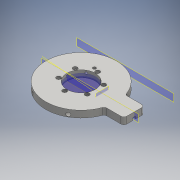
# Autodesk Inventor part: top
Saved by Autodesk Inventor 2016 (Build 200138000, 138)
## iProperties
Created: 2017-05-24
Part Number: top
Material: Generic
Document SubType Name: Modeling
Designer: bitbots
Density: 1 g/cm^3
Appearance: Default
Author: bitbots
Autodesk Inventor part; units mm, degrees
ref_plane "YZ Plane" through (0, 0, 0) normal (1, 0, 0) x (0, 1, 0)
ref_plane "XZ Plane" through (0, 0, 0) normal (0, 1, 0) x (-1, 0, 0)
ref_plane "XY Plane" through (0, 0, 0) normal (0, 0, 1) x (1, 0, 0)
ref_plane "Work Plane1" through (0, 0, 0) normal (0, 0, 1) x (1, 0, 0)
sketch "Sketch1" plane through (0, 0, 0) normal (0, 0, 1) x (1, 0, 0)
  circle A0 centre (7.7356, -42.5713) radius 1.65 construction
  circle A1 centre (7.7356, -14.5713) radius 1.65 construction
  circle A2 centre (-40.7618, -14.5713) radius 1.65 construction
  circle A3 centre (-40.7618, -42.5713) radius 1.65 construction
  circle A4 centre (-16.5131, -56.5713) radius 1.65 construction
  circle A5 centre (-16.5131, -28.5713) radius 23 construction
  circle A6 centre (-16.5131, -0.5713) radius 1.65 construction
  line L0 (8.9285, -4.5354) -> (9.6603, -3.2679) construction
  line L1 (9.6603, -3.2679) -> (-7.1349, 6.4287) construction
  line L2 (-7.1349, 6.4287) -> (-7.8354, 6.4287) construction
  line L3 (-7.8354, 6.4287) -> (-8.3875, 5.4724) construction
  arc A7 (-8.3875, 5.4724) -> (-45.0507, -8.3079) centre (-16.5131, -28.5713) ccw construction
  line L4 (-45.0507, -8.3079) -> (-48.3766, -7.7215) construction
  line L5 (-48.3766, -7.7215) -> (-53.5861, -37.2657) construction
  line L6 (-53.5861, -37.2657) -> (-50.2602, -37.8522) construction
  arc A8 (-50.2602, -37.8522) -> (-45.3149, -48.4574) centre (-16.5131, -28.5713) ccw construction
  line L7 (-45.3149, -48.4574) -> (-47.0035, -51.3822) construction
  line L8 (-47.0035, -51.3822) -> (-25.3528, -63.8822) construction
  line L9 (-25.3528, -63.8822) -> (-24.6234, -62.6186) construction
  arc A9 (-24.6234, -62.6186) -> (8.9285, -4.5354) centre (-16.5131, -28.5713) ccw construction
  circle A10 centre (-16.5131, -28.5713) radius 23
  circle A11 centre (-16.5131, -28.5713) radius 35
  circle A12 centre (-16.5131, -56.5713) radius 1.65
  circle A13 centre (-40.7618, -42.5713) radius 1.65
  circle A14 centre (-40.7618, -14.5713) radius 1.65
  circle A15 centre (-16.5131, -0.5713) radius 1.65
  circle A16 centre (7.7356, -14.5713) radius 1.65
  circle A17 centre (7.7356, -42.5713) radius 1.65
  point P0 (0, 0)
  constraints: 8 centre point, 8 coincident, 8 concentric
extrude "Extrusion1" add sketch "Sketch1" along normal blind 11.5
ref_plane "Work Plane2" through (18.4869, -28.5713, 6.2613) normal (-0.9961947, 0, 0.0871557) x (0, -1, 0)
sketch "Sketch2" plane through (18.4869, -28.5713, 6.2613) normal (-0.9961947, 0, 0.0871557) x (0, -1, 0)
  spline S0 degree 3 poles (-1.3526, 0) (-1.3526, 0.1694) (-1.3188, 0.3504) (-1.1809, 0.6837) (-1.0768, 0.836) (-0.8365, 1.0764) (-0.6844, 1.1805) (-0.3511, 1.3186) (-0.1699, 1.3526) (0.1699, 1.3526) (0.3511, 1.3186) (0.6844, 1.1805) (0.8365, 1.0764) (1.0768, 0.836) (1.1809, 0.6837) (1.3188, 0.3504) (1.3525, 0.1694) (1.3525, -0.1702) (1.3185, -0.3514) (1.1804, -0.6845) (1.0764, -0.8364) (0.8367, -1.0761) (0.685, -1.1801) (0.3518, -1.3184) (0.1704, -1.3525) (-0.1704, -1.3525) (-0.3518, -1.3184) (-0.685, -1.1801) (-0.8367, -1.0761) (-1.0764, -0.8364) (-1.1804, -0.6845) (-1.3185, -0.3514) (-1.3526, -0.1702) (-1.3526, 0) knots 0 0 0 0 0.05101 0.05101 0.10202 0.10202 0.152982 0.152982 0.203944 0.203944 0.254906 0.254906 0.305868 0.305868 0.356878 0.356878 0.407888 0.407888 0.459155 0.459155 0.510422 0.510422 0.561534 0.561534 0.612646 0.612646 0.663758 0.663758 0.71487 0.71487 0.766137 0.766137 0.817404 0.817404 0.817404 0.817404 construction
  circle A0 centre (0, 0) radius 1.8
  point P0 (-28.5713, -7.8487)
  point P1 (-1.3526, 0)
  dimension "d2" = 3.6
  constraints: 1 centre point
  measures "d2" diameter of A0
extrude "Extrusion2" cut sketch "Sketch2" along normal mid plane 30
sketch "Sketch3" plane through (18.4869, -28.5713, 6.2613) normal (-0.9961947, 0, 0.0871557) x (0, -1, 0)
  spline S0 degree 2 poles (1.8, 0) (1.8, 3.1177) (-0.9, 1.5588) (-3.6, 0) (-0.9, -1.5588) (1.8, -3.1177) (1.8, 0) knots 0 0 0 0.333333 0.333333 0.666667 0.666667 1 1 1 weights 1 0.5 1 0.5 1 0.5 1 projected
  circle A0 centre (0, 0) radius 3.15
  point P0 (-28.5713, -7.8487)
  dimension "d5" = 6.3
  constraints: 1 centre point, 1 other
  measures "d5" diameter of A0
extrude "Extrusion3" cut sketch "Sketch3" along normal mid plane 6
pattern_circular "Circular Pattern1" count 6 over 360 about axis through (-16.5131, -28.5713, 0) along (0, 0, 1) of "Extrusion3", "Extrusion2"
ref_plane "Work Plane3" through (-16.5131, -28.5713, 2.5) normal (0, 0, -1) x (-1, 0, 0)
sketch "Sketch4" plane through (-16.5131, -28.5713, 2.5) normal (0, 0, -1) x (-1, 0, 0)
  line L0 (2.7846, -43.1769) -> (-38.7846, -19.1769) projected
  line L1 (2.7846, -43.1769) -> (-5.2154, -57.0333) projected
  line L2 (-46.7846, -33.0333) -> (-5.2154, -57.0333) projected
  line L3 (-38.7846, -19.1769) -> (-46.7846, -33.0333) projected
  circle A0 centre (0, 0) radius 35 projected
  line L4 (2.7846, -43.1769) -> (8.0469, -34.0624)
  line L5 (-38.7846, -19.1769) -> (-33.5223, -10.0624)
  line L6 (8.0469, -34.0624) -> (-17.5, -30.3109)
  line L7 (-17.5, -30.3109) -> (-33.5223, -10.0624)
  point P0 (-16.5131, 28.5713)
  constraints: 8 end point, 3 point on circle, 1 parallel
extrude "Extrusion4" add sketch "Sketch4" against normal blind 2 contours L1 L2 L3 L0 | L0 L5 A0 L4
ref_plane "Work Plane4" through (-16.5131, -28.5713, 7) normal (0, 0, -1) x (-1, 0, 0)
sketch "Sketch5" plane through (-16.5131, -28.5713, 7) normal (0, 0, -1) x (-1, 0, 0)
  line L0 (-36, -4) -> (-87, -4) projected
  line L1 (-36, -4) -> (-36, -14) projected
  line L2 (-87, -14) -> (-36, -14) projected
  line L3 (-87, -4) -> (-87, -14) projected
  line L4 (8.0469, -34.0624) -> (-5.2154, -57.0333) projected
  line L5 (-5.2154, -57.0333) -> (-46.7846, -33.0333) projected
  line L6 (-46.7846, -33.0333) -> (-33.5223, -10.0624) projected
  arc A0 (-33.5223, -10.0624) -> (-19.7119, -28.9213) centre (0, 0) ccw projected
  arc A1 (-19.7119, -28.9213) -> (-15.1906, -31.5317) centre (0, 0) ccw projected
  arc A2 (-15.1906, -31.5317) -> (8.0469, -34.0624) centre (0, 0) ccw projected
  circle A3 centre (0, 0) radius 35 projected
  line L7 (-87, -4) -> (-87, 0)
  line L8 (29.1046, -46.4106) -> (37.7648, -41.4106) projected
  line L9 (38.7648, -43.1426) -> (37.7648, -41.4106) projected
  arc A4 (38.7648, -43.1426) -> (58, 0.0727) centre (0, 0) ccw projected
  line L10 (58, 0.0727) -> (56.0303, -0.2746) projected
  line L11 (56.0303, -0.2746) -> (52.5574, 19.4215) projected
  line L12 (54.527, 19.7688) -> (52.5574, 19.4215) projected
  arc A5 (54.527, 19.7688) -> (11.225, 56.9034) centre (0, 0) ccw projected
  line L13 (11.225, 58.9406) -> (11.225, 56.9034) projected
  arc A6 (-56.2907, -20.7692) -> (11.225, 58.9406) centre (0, 0) ccw construction
  arc A7 (-56.2907, -20.7692) -> (-60.9816, -17.5) centre (-60.9816, -22.5) ccw projected
  line L14 (-85, -17.5) -> (-60.9816, -17.5) projected
  arc A8 (-90, -12.5) -> (-85, -17.5) centre (-85, -12.5) ccw projected
  line L15 (-90, 0) -> (-90, -12.5) projected
  line L16 (-88, 0) -> (-90, 0) projected
  line L17 (-88, -10.5) -> (-88, 0) projected
  arc A9 (-88, -10.5) -> (-83, -15.5) centre (-83, -10.5) ccw projected
  line L18 (-42.5, -15.5) -> (-83, -15.5) projected
  line L19 (-42.5, -15.5) -> (-42.5, -19.5) projected
  line L20 (-42.5, -19.5) -> (-54.6237, -19.5) projected
  arc A10 (-54.6237, -19.5) -> (-51.3747, -26.9191) centre (0, 0) ccw projected
  line L21 (-51.3747, -26.9191) -> (-45.7176, -30.1852) projected
  line L22 (-45.7176, -30.1852) -> (-47.2176, -32.7833) projected
  line L23 (-47.2176, -32.7833) -> (-4.7824, -57.2833) projected
  line L24 (-4.7824, -57.2833) -> (-3.2824, -54.6852) projected
  line L25 (-3.2824, -54.6852) -> (2.3747, -57.9514) projected
  arc A11 (2.3747, -57.9514) -> (30.7148, -49.1996) centre (0, 0) ccw projected
  line L26 (30.7148, -49.1996) -> (29.1046, -46.4106) projected
  line L27 (-60.9816, -17.5) -> (-60.9816, -15.5)
  line L28 (-60.9816, -15.5) -> (-83, -15.5)
  line L29 (-90, 0) -> (-87, 0)
  line L30 (-87, -4) -> (-90, -4)
  line L31 (-90, -4) -> (-90, 0)
  line L32 (-88, -4) -> (-29.7606, -4)
  line L33 (-29.7606, -4) -> (-29.7606, -15.5)
  line L34 (-29.7606, -15.5) -> (-88, -15.5)
  line L35 (-88, -15.5) -> (-88, -4)
  line L36 (-54.6237, -19.5) -> (-35.2604, -19.5)
  line L37 (-35.2604, -19.5) -> (-35.2604, -15.5)
  line L38 (-35.2604, -15.5) -> (-54.6237, -15.5)
  line L39 (-54.6237, -15.5) -> (-54.6237, -19.5)
  line L40 (-47.9586, -33.5041) -> (-35.2604, -33.5041)
  line L41 (-35.2604, -33.5041) -> (-35.2604, -19.5)
  line L42 (-35.2604, -19.5) -> (-47.9586, -19.5)
  line L43 (-47.9586, -19.5) -> (-47.9586, -33.5041)
  line L44 (-47.9586, -19.5) -> (-51.9058, -19.5)
  line L45 (-51.9058, -19.5) -> (-51.9058, -28.939)
  line L46 (-51.9058, -28.939) -> (-47.9586, -28.939)
  line L47 (-47.9586, -28.939) -> (-47.9586, -19.5)
  line L48 (-51.9058, -19.5) -> (-53.3897, -19.5)
  line L49 (-53.3897, -19.5) -> (-53.3897, -26.2863)
  line L50 (-53.3897, -26.2863) -> (-51.9058, -26.2863)
  line L51 (-51.9058, -26.2863) -> (-51.9058, -19.5)
  line L52 (-53.3897, -19.5) -> (-55.0309, -19.5)
  line L53 (-55.0309, -19.5) -> (-55.0309, -22.8932)
  line L54 (-55.0309, -22.8932) -> (-53.3897, -22.8932)
  line L55 (-53.3897, -22.8932) -> (-53.3897, -19.5)
  line L56 (-3.2824, -54.6852) -> (8.7201, -33.8963)
  line L57 (8.7201, -33.8963) -> (8.4423, -33.3775)
  line L58 (8.0469, -34.0624) -> (-5.2154, -57.0333) projected
  line L59 (8.4423, -33.3775) -> (8.0469, -34.0624)
  line L60 (8.0469, -34.0624) -> (-5.2154, -57.0333)
  line L61 (-5.2154, -57.0333) -> (-4.7824, -57.2833)
  line L62 (-3.2824, -54.6852) -> (-4.7824, -57.2833)
  line L63 (-4.7824, -57.2833) -> (-6.1674, -59.6822)
  arc A12 (-56.2907, -20.7692) -> (-6.1674, -59.6822) centre (0, 0) ccw
  line L64 (-47.2176, -32.7833) -> (-47.2176, -21.5468)
  line L65 (-47.2176, -21.5468) -> (-54.6237, -15.5)
  line L66 (-54.6237, -15.5) -> (-60.9816, -15.5)
  point P0 (-16.5131, 28.5713)
  dimension "d15" = 4
  constraints: 80 end point, 13 parallel, 11 perpendicular, 7 point on line, 6 horizontal, 4 point on circle, 3 collinear, 1 centre point, 1 coincident, 1 tangent, 1 vertical
  measures "d15" distance of L0.end L7.end
extrude "Extrusion5" add sketch "Sketch5" against normal blind 2 contours L1 L2 A9 L3 L0 | L32 A3 L6 L34 L18 A9 L2 L1 | L3 A9 L17 L30 | L32 L33 L34 A0 A3 | A9 L2 L3 | L3 L2 A9 L34 L35 | L17 L35 L34 L18 L27 L14 A8 L15 L30 | A0 L34 L6 | L56 L24 L23 L4 A3 | A3 L59 L57 | L34 L37 L36 L6 | L6 L36 L19 L34 | A0 A1 A2 L4 L5 L40 L41 L37 L34 | L18 L39 L52 L53 L54 L49 L50 L45 L46 L43 L40 L5 L23 L63 A12 A7 L27 | L36 L41 L40 L5 L6 | L6 L23 L22 L21 L64 L65 L43 L20 L36 | L19 L20 L65 L18 | L65 L20 L39 | L5 L40 L43 L21 L64 L23 | L20 L49 A10 | A10 L49 L54 L53 L52 | L65 L43 L21 A10 L45 L20 | L20 L43 L65 | L64 L21 L22 | L20 L45 A10 L49 | A10 L45 L50 L49 | L65 L64 L21 L43 | A10 L21 L43 L46 L45
sketch "Sketch6" plane through (-16.5131, -28.5713, 4.5) normal (0, 0, 1) x (1, 0, 0)
  line L0 (-8.0469, -34.0624) -> (5.2154, -57.0333) projected
  line L1 (5.2154, -57.0333) -> (46.7846, -33.0333) projected
  line L2 (46.7846, -33.0333) -> (33.5223, -10.0624) projected
  arc A0 (19.7119, -28.9213) -> (33.5223, -10.0624) centre (0, 0) ccw projected
  arc A1 (15.1906, -31.5317) -> (19.7119, -28.9213) centre (0, 0) ccw projected
  arc A2 (-8.0469, -34.0624) -> (15.1906, -31.5317) centre (0, 0) ccw projected
  point P0 (16.5131, 28.5713)
extrude "Extrusion6" add sketch "Sketch6" along normal up to surface (2.5 mm away)
sketch "Sketch7" plane through (-16.5131, -28.5713, 11.5) normal (0, 0, 1) x (1, 0, 0)
  arc A0 (-11.225, 58.9406) -> (56.2907, -20.7692) centre (0, 0) ccw construction
  arc A1 (-8.7201, -33.8963) -> (34.7707, -4) centre (0, 0) ccw projected
  circle A2 centre (0, 0) radius 35
  arc A3 (90, 12.5) -> (85, 17.5) centre (85, 12.5) ccw projected
  line L0 (90, 12.5) -> (90, -12.5) projected
  arc A4 (85, -17.5) -> (90, -12.5) centre (85, -12.5) ccw projected
  line L1 (85, -17.5) -> (60.9816, -17.5) projected
  arc A5 (60.9816, -17.5) -> (56.2907, -20.7692) centre (60.9816, -22.5) ccw projected
  arc A6 (56.2907, 20.7692) -> (56.2907, -20.7692) centre (0, 0) ccw construction
  arc A7 (56.2907, 20.7692) -> (60.9816, 17.5) centre (60.9816, 22.5) ccw projected
  line L2 (60.9816, 17.5) -> (85, 17.5) projected
  circle A8 centre (0, 0) radius 33 construction
  arc A9 (56.2907, 20.7692) -> (56.2907, -20.7692) centre (0, 0) ccw
  point P0 (16.5131, 28.5713)
  constraints: 2 centre point, 2 coincident, 2 point on circle
extrude "Extrusion7" add sketch "Sketch7" against normal up to surface (4.5 mm away)
sketch "Sketch8" plane through (0, 0, 11.5) normal (0, 0, 1) x (1, 0, 0)
  circle A0 centre (7.7356, -42.5713) radius 1.65 projected
  circle A1 centre (7.7356, -42.5713) radius 3.1
  arc A2 (-47.8124, -39.0285) -> (15.6233, -36.0713) centre (-16.5131, -28.5713) ccw projected
  arc A3 (44.4685, -46.0713) -> (39.7776, -49.3405) centre (44.4685, -51.0713) ccw projected
  line L0 (44.4685, -46.0713) -> (68.4869, -46.0713) projected
  arc A4 (68.4869, -46.0713) -> (73.4869, -41.0713) centre (68.4869, -41.0713) ccw projected
  line L1 (73.4869, -41.0713) -> (73.4869, -16.0713) projected
  arc A5 (73.4869, -16.0713) -> (68.4869, -11.0713) centre (68.4869, -16.0713) ccw projected
  line L2 (68.4869, -11.0713) -> (44.4685, -11.0713) projected
  arc A6 (39.7776, -7.802) -> (44.4685, -11.0713) centre (44.4685, -6.0713) ccw projected
  arc A7 (39.7776, -7.802) -> (39.7776, -49.3405) centre (-16.5131, -28.5713) ccw projected
  circle A8 centre (-16.5131, -28.5713) radius 23 projected
  circle A9 centre (7.7356, -42.5713) radius 1.65 projected
  circle A10 centre (7.7356, -14.5713) radius 1.65 projected
  circle A11 centre (-16.5131, -0.5713) radius 1.65 projected
  circle A12 centre (-40.7618, -14.5713) radius 1.65 projected
  circle A13 centre (-40.7618, -42.5713) radius 1.65 projected
  circle A14 centre (-16.5131, -56.5713) radius 1.65 projected
  circle A15 centre (7.7356, -14.5713) radius 3.1
  circle A16 centre (-16.5131, -0.5713) radius 3.1
  circle A17 centre (-40.7618, -14.5713) radius 3.1
  circle A18 centre (-40.7618, -42.5713) radius 3.1
  circle A19 centre (-16.5131, -56.5713) radius 3.1
  point P0 (0, 0)
  dimension "d22" = 6.2
  dimension "d25" = 360
  constraints: 6 centre point, 1 coincident, 13 other
  measures "d22" diameter of A1
extrude "Extrusion8" cut sketch "Sketch8" against normal blind 3.5 contours A1 | A10 | A15 | A16 | A17 | A18 | A19
sketch "Sketch9" plane through (-16.5131, -28.5713, 7) normal (0, 0, -1) x (-1, 0, 0)
  line L0 (-90, 12.5) -> (-90, -12.5) construction
  arc A0 (-90, -12.5) -> (-85, -17.5) centre (-85, -12.5) ccw construction
  line L1 (-85, -17.5) -> (-60.9816, -17.5) construction
  arc A1 (-56.2907, -20.7692) -> (-60.9816, -17.5) centre (-60.9816, -22.5) ccw construction
  arc A2 (-56.2907, -20.7692) -> (-56.2907, 20.7692) centre (0, 0) ccw construction
  arc A3 (-60.9816, 17.5) -> (-56.2907, 20.7692) centre (-60.9816, 22.5) ccw construction
  line L2 (-60.9816, 17.5) -> (-85, 17.5) projected
  arc A4 (-85, 17.5) -> (-90, 12.5) centre (-85, 12.5) ccw projected
  arc A5 (-34.8655, -3.0656) -> (-33.5223, -10.0624) centre (0, 0) ccw construction
  arc A6 (-34.8655, 3.0656) -> (-34.8655, -3.0656) centre (0, 0) ccw construction
  arc A7 (-20.0876, 28.6616) -> (-34.8655, 3.0656) centre (0, 0) ccw construction
  arc A8 (-14.7778, 31.7272) -> (-20.0876, 28.6616) centre (0, 0) ccw construction
  arc A9 (14.7778, 31.7272) -> (-14.7778, 31.7272) centre (0, 0) ccw construction
  arc A10 (20.0876, 28.6616) -> (14.7778, 31.7272) centre (0, 0) ccw construction
  arc A11 (34.8655, 3.0656) -> (20.0876, 28.6616) centre (0, 0) ccw construction
  arc A12 (34.8655, -3.0656) -> (34.8655, 3.0656) centre (0, 0) ccw construction
  arc A13 (20.0876, -28.6616) -> (34.8655, -3.0656) centre (0, 0) ccw construction
  arc A14 (14.7778, -31.7272) -> (20.0876, -28.6616) centre (0, 0) ccw construction
  arc A15 (8.0469, -34.0624) -> (14.7778, -31.7272) centre (0, 0) ccw construction
  line L3 (8.0469, -34.0624) -> (-5.2154, -57.0333) construction
  line L4 (-5.2154, -57.0333) -> (-46.7846, -33.0333) construction
  line L5 (-46.7846, -33.0333) -> (-33.5223, -10.0624) construction
  line L6 (-90, -12.5) -> (-90, 12.5) projected
  line L7 (-90, 0) -> (-35, 0)
  circle A16 centre (0, 0) radius 35 projected
  line L8 (8.0469, -34.0624) -> (8.0469, -59.458)
  arc A17 (-56.2907, -20.7692) -> (-56.2907, 20.7692) centre (0, 0) ccw projected
  line L9 (8.0469, -34.0624) -> (33.4424, -34.0624) construction
  arc A18 (8.0469, -34.0624) -> (-35, 0) centre (0, 0) ccw
  arc A19 (-60.9816, 17.5) -> (-56.2907, 20.7692) centre (-60.9816, 22.5) ccw projected
  arc A20 (8.0469, -59.458) -> (-56.2907, 20.7692) centre (0, 0) ccw
  line L10 (-90, 12.5) -> (-90, -12.5) projected
  line L11 (-90, 0) -> (-90, 12.5)
  line L12 (-5.2154, -57.0333) -> (8.0469, -34.0624) projected
  arc A21 (-33.5223, -10.0624) -> (8.0469, -34.0624) centre (0, 0) ccw projected
  line L13 (-33.5223, -10.0624) -> (-46.7846, -33.0333) projected
  line L14 (-46.7846, -33.0333) -> (-5.2154, -57.0333) projected
  line L15 (-46.7846, -33.0333) -> (-5.2154, -57.0333) projected
  line L16 (-46.7846, -33.0333) -> (-48.2801, -35.6235)
  arc A22 (-56.2907, -20.7692) -> (-56.2907, 20.7692) centre (0, 0) ccw projected
  line L17 (-46.7846, -33.0333) -> (-43.7937, -33.0333) construction
  arc A23 (-48.2801, -35.6235) -> (8.0469, -59.458) centre (0, 0) ccw
  line L18 (-5.2154, -57.0333) -> (8.0469, -34.0624) projected
  line L19 (-46.7846, -33.0333) -> (-5.2154, -57.0333)
  line L20 (-5.2154, -57.0333) -> (8.0469, -34.0624)
  arc A24 (-48.2801, -35.6235) -> (8.0469, -59.458) centre (0, 0) ccw
  line L21 (-48.2801, -35.6235) -> (-46.7846, -33.0333)
  line L22 (-46.7846, -33.0333) -> (-5.2154, -57.0333)
  line L23 (-5.2154, -57.0333) -> (8.0469, -34.0624)
  point P0 (-16.5131, 28.5713)
  dimension "d29" = 90
  dimension "d32" = 120
  constraints: 22 end point, 11 point on circle, 4 centre point, 4 coincident, 2 collinear, 2 equal length, 2 horizontal, 2 perpendicular, 1 midpoint, 1 vertical, 2 other
  measures "d29" angle of L8 L9
  measures "d32" angle of L16 L17
extrude "Extrusion9" add sketch "Sketch9" along normal blind 7 contours A19 A17 L8 A16 L7 L6 A4 L2 | A17 L16 L14 L12 L8
sketch "Sketch10" plane through (0, 0, 0) normal (0, 0, -1) x (-1, 0, 0)
  line L0 (-31.767, -64.1948) -> (-17.0093, -38.6337) construction
  arc A0 (-18.3524, -31.6369) -> (-17.0093, -38.6337) centre (16.5131, -28.5713) ccw construction
  arc A1 (-18.4869, -28.5713) -> (-18.3524, -31.6369) centre (16.5131, -28.5713) ccw construction
  line L1 (-18.4869, -28.5713) -> (-73.4869, -28.5713) construction
  line L2 (-73.4869, -28.5713) -> (-73.4869, -41.0713) projected
  arc A2 (-73.4869, -41.0713) -> (-68.4869, -46.0713) centre (-68.4869, -41.0713) ccw projected
  line L3 (-68.4869, -46.0713) -> (-44.4685, -46.0713) projected
  arc A3 (-39.7776, -49.3405) -> (-44.4685, -46.0713) centre (-44.4685, -51.0713) ccw projected
  arc A4 (-39.7776, -49.3405) -> (-31.767, -64.1948) centre (16.5131, -28.5713) ccw projected
  line L4 (11.2977, -85.6046) -> (-30.2715, -61.6046) construction
  line L5 (-30.2715, -61.6046) -> (-31.767, -64.1948) projected
  line L6 (-31.767, -64.1948) -> (-30.2715, -61.6046)
  line L7 (-73.4869, -28.5713) -> (-71.4869, -28.5713)
  line L8 (-71.4869, -28.5713) -> (-71.4869, -41.2625)
  line L9 (-44.4685, -46.0713) -> (-68.4869, -46.0713) projected
  line L10 (-68.4869, -46.0713) -> (-68.4869, -44.0713)
  line L11 (-68.4869, -44.0713) -> (-71.4869, -41.2625)
  arc A5 (-38.6208, -44.0713) -> (-30.2715, -61.6046) centre (16.5131, -28.5713) ccw
  line L12 (-38.6208, -44.0713) -> (-68.4869, -44.0713)
  point P0 (0, 0)
  dimension "d33" = 2
  dimension "d34" = 2
  constraints: 12 end point, 2 point on circle, 1 centre point, 1 coincident, 1 collinear, 1 horizontal, 1 perpendicular, 1 point on line, 1 vertical
  measures "d33" distance of L1.end L7.end
  measures "d34" distance of L3.start L10.end
extrude "Extrusion10" add sketch "Sketch10" against normal up to surface (7 mm away)
sketch "Sketch11" plane through (15.4983, -28.5713, 6.5227) normal (0.9961947, 0, -0.0871557) x (-0.0871557, 0, -0.9961947)
  circle A0 centre (0, 0) radius 1.8 projected
  circle A1 centre (0, 0) radius 3.15 projected
  point P0 (7.8487, 28.5713)
extrude "Extrusion11" cut sketch "Sketch11" along normal blind 100 contours A0 | A1
pattern_circular "Circular Pattern2" count 6 over 360 about axis through (-16.5131, -28.5713, 0) along (0, 0, 1) of "Extrusion11"
ref_plane "Work Plane6" through (44.4685, 31.4287, 11.5) normal (0, 1, 0) x (1, 0, 0)
ref_plane "Work Plane5" through (44.4685, -28.5713, 11.5) normal (0, 1, 0) x (1, 0, 0)
sketch "Sketch12" plane through (44.4685, 31.4287, 11.5) normal (0, 1, 0) x (1, 0, 0)
  spline S0 degree 3 poles (-73.4816, 17) (-73.4816, 18.5746) (-73.1659, 20.2508) (-71.8889, 23.3291) (-70.9276, 24.7316) (-68.7132, 26.946) (-67.3107, 27.9073) (-64.2323, 29.1844) (-62.556, 29.5) (-59.4071, 29.5) (-57.7308, 29.1844) (-54.6524, 27.9073) (-53.2499, 26.946) (-51.0355, 24.7316) (-50.0743, 23.3291) (-48.7972, 20.2508) (-48.4816, 18.5746) (-48.4816, 15.4254) (-48.7972, 13.7492) (-49.5353, 11.97) (-49.6424, 11.733) (-49.7566, 11.5) knots 0 0 0 0 0.472366 0.472366 0.944732 0.944732 1.417066 1.417066 1.8894 1.8894 2.361735 2.361735 2.834069 2.834069 3.306435 3.306435 3.778801 3.778801 4.251167 4.251167 4.324846 4.324846 4.324846 4.324846 projected
  spline S1 degree 3 poles (-72.2065, 11.5) (-72.3207, 11.733) (-72.4278, 11.97) (-73.1659, 13.7492) (-73.4816, 15.4254) (-73.4816, 17) knots 7.011557 7.011557 7.011557 7.011557 7.085236 7.085236 7.557602 7.557602 7.557602 7.557602 projected
  line L0 (-120.9816, 0) -> (-4.6909, 0) construction
  line L1 (-4.6909, 11.5) -> (-120.9816, 11.5) construction
  line L2 (-37.9816, 0) -> (-83.9816, 0) construction
  line L3 (-60.9816, 0) -> (-60.9816, 17) construction
  line L4 (-60.9816, 0) -> (-43.9816, 0) construction
  circle A0 centre (-60.9816, 17) radius 12.4991
  point P0 (-44.4685, 11.5)
  dimension "d43" = 17
  dimension "d44" = 90
  constraints: 4 end point, 1 centre point, 1 coincident, 1 horizontal, 1 midpoint, 1 perpendicular, 1 vertical
  measures "d43" distance of L3.start L3.end
  measures "d44" angle of L4 L3
extrude "Extrusion12" cut sketch "Sketch12" against normal blind 10
sketch "Sketch13" plane through (0, 0, 11.5) normal (0, 0, 1) x (1, 0, 0)
  circle A0 centre (-24.7306, 2.0969) radius 2.3939 construction
  circle A1 centre (-24.7306, 2.0969) radius 2.6
  point P0 (0, 0)
  dimension "d47" = 5.2
  constraints: 1 centre point, 1 coincident
  measures "d47" diameter of A1
extrude "Extrusion13" cut sketch "Sketch13" against normal blind 10
sketch "Sketch14" plane through (0, 0, 0) normal (0, 0, -1) x (-1, 0, 0)
  circle A0 centre (40.7618, -14.5713) radius 1.65 construction
  circle A1 centre (40.7618, -14.5713) radius 2.15
  point P0 (0, 0)
  dimension "d50" = 4.3
  constraints: 1 centre point, 1 coincident
  measures "d50" diameter of A1
extrude "Extrusion14" cut sketch "Sketch14" against normal through all
pattern_circular "Circular Pattern3" count 6 over 360 about axis through (-16.5131, -28.5713, 0) along (0, 0, 1) of "Extrusion14"
sketch "Sketch15" plane through (0, 0, 11.5) normal (0, 0, 1) x (1, 0, 0)
  circle A0 centre (-40.7618, -14.5713) radius 3.1 projected
  circle A1 centre (-40.7618, -14.5713) radius 3.65
  point P0 (0, 0)
  dimension "d56" = 7.3
  constraints: 1 centre point, 1 coincident
  measures "d56" diameter of A1
extrude "Extrusion15" cut sketch "Sketch15" against normal up to surface (3.5 mm away)
pattern_circular "Circular Pattern4" count 6 over 360 about axis through (-16.5131, -28.5713, 0) along (0, 0, 1) of "Extrusion15"
sketch "Sketch17" plane through (0, 0, 0) normal (0, 0, -1) x (-1, 0, 0)
  circle A0 centre (16.5131, -0.5713) radius 2.15 projected
  circle A1 centre (-7.7356, -14.5713) radius 2.15 projected
  circle A2 centre (-7.7356, -42.5713) radius 2.15 projected
  circle A3 centre (16.5131, -56.5713) radius 2.15 projected
  circle A4 centre (40.7618, -42.5713) radius 2.15 projected
  circle A5 centre (40.7618, -14.5713) radius 2.15 projected
  circle A6 centre (16.5131, -28.5713) radius 23 projected
  line L0 (27.7371, 30.3696) -> (27.7371, 21.4287) projected
  line L1 (27.7371, 21.4287) -> (5.2891, 21.4287) projected
  line L2 (5.2891, 21.4287) -> (5.2891, 30.3696) projected
  arc A7 (5.2891, 30.3696) -> (-39.7776, -7.802) centre (16.5131, -28.5713) ccw projected
  arc A8 (-44.4685, -11.0713) -> (-39.7776, -7.802) centre (-44.4685, -6.0713) ccw projected
  line L3 (-44.4685, -11.0713) -> (-68.4869, -11.0713) projected
  arc A9 (-68.4869, -11.0713) -> (-73.4869, -16.0713) centre (-68.4869, -16.0713) ccw projected
  line L4 (-73.4869, -16.0713) -> (-73.4869, -25.7717) projected
  ellipse E0 centre (-90.0533, -28.5713) end of major axis (-126.1955, -28.5713) minor radius 3.15 (-53.9112, -28.5713) -> (-73.4869, -25.7717) ccw projected
  line L5 (-53.9112, -28.5713) -> (-18.4869, -28.5713) projected
  arc A10 (-18.4869, -28.5713) -> (24.56, -62.6337) centre (16.5131, -28.5713) ccw projected
  line L6 (24.56, -62.6337) -> (11.2977, -85.6046) projected
  line L7 (11.2977, -85.6046) -> (-30.2715, -61.6046) projected
  arc A11 (-38.6208, -44.0713) -> (-30.2715, -61.6046) centre (16.5131, -28.5713) ccw projected
  line L8 (-38.6208, -44.0713) -> (-68.4869, -44.0713) projected
  line L9 (-68.4869, -44.0713) -> (-71.4869, -41.2625) projected
  line L10 (-71.4869, -41.2625) -> (-71.4869, -31.2739) projected
  ellipse E1 centre (-90.0533, -28.5713) end of major axis (-126.1955, -28.5713) minor radius 3.15 (-73.4869, -31.3709) -> (-71.4869, -31.2739) ccw projected
  line L11 (-73.4869, -31.3709) -> (-73.4869, -41.0713) projected
  arc A12 (-73.4869, -41.0713) -> (-68.4869, -46.0713) centre (-68.4869, -41.0713) ccw projected
  line L12 (-68.4869, -46.0713) -> (-44.4685, -46.0713) projected
  arc A13 (-39.7776, -49.3405) -> (-44.4685, -46.0713) centre (-44.4685, -51.0713) ccw projected
  arc A14 (-39.7776, -49.3405) -> (27.7371, 30.3696) centre (16.5131, -28.5713) ccw projected
  arc A15 (-39.7776, -49.3405) -> (-39.7776, -7.802) centre (16.5131, -28.5713) ccw projected
  arc A16 (45.5131, 21.6582) -> (16.5131, 29.4287) centre (16.5131, -28.5713) ccw
  line L13 (16.5131, -28.5713) -> (16.5131, 29.4287) construction
  line L14 (16.5131, -28.5713) -> (74.5131, -28.5713) construction
  line L15 (16.5131, -28.5713) -> (45.5131, 21.6582) construction
  arc A17 (16.5131, 29.4287) -> (-12.4869, 21.6582) centre (16.5131, -28.5713) ccw
  line L16 (16.5131, -28.5713) -> (-12.4869, 21.6582) construction
  line L17 (16.5131, -28.5713) -> (16.5131, 29.4287) construction
  arc A18 (41.5131, 14.73) -> (16.5131, 21.4287) centre (16.5131, -28.5713) ccw
  line L18 (16.5131, -28.5713) -> (16.5131, 21.4287) construction
  line L19 (16.5131, -28.5713) -> (66.5131, -28.5713) construction
  arc A19 (16.5131, 21.4287) -> (-8.4869, 14.73) centre (16.5131, -28.5713) ccw
  line L20 (16.5131, -28.5713) -> (-8.4869, 14.73) construction
  line L21 (16.5131, -28.5713) -> (16.5131, 21.4287) construction
  line L22 (45.5131, 21.6582) -> (41.5131, 14.73)
  line L23 (-8.4869, 14.73) -> (-12.4869, 21.6582)
  dimension "d72" = 58
  dimension "d73" = 90
  dimension "d74" = 30
  dimension "d75" = 30
  dimension "d76" = 50
  dimension "d77" = 90
  dimension "d78" = 30
  constraints: 22 end point, 8 point on circle, 4 centre point, 4 coincident, 2 horizontal, 2 perpendicular, 1 collinear, 2 other
  measures "d72" radius of A16
  measures "d73" angle of L14 L13
  measures "d74" angle of L15 L13
  measures "d75" angle of L17 L16
  measures "d76" radius of A18
  measures "d77" angle of L19 L18
  measures "d78" angle of L21 L20
extrude "Extrusion17" cut sketch "Sketch17" against normal blind 9.5 contours A16 L22 A18 L1 L0 | L0 L1 L2 A17 A16 | L2 L1 A19 L23 A17
sketch "Sketch16" plane through (0, 0, 0) normal (0, 0, -1) x (-1, 0, 0)
  circle A0 centre (16.5131, -0.5713) radius 2.15 projected
  circle A1 centre (-7.7356, -14.5713) radius 2.15 projected
  circle A2 centre (-7.7356, -42.5713) radius 2.15 projected
  circle A3 centre (16.5131, -56.5713) radius 2.15 projected
  circle A4 centre (40.7618, -42.5713) radius 2.15 projected
  circle A5 centre (40.7618, -14.5713) radius 2.15 projected
  circle A6 centre (16.5131, -28.5713) radius 23 projected
  line L0 (27.7371, 30.3696) -> (27.7371, 28.3323) projected
  line L1 (5.2891, 28.3323) -> (5.2891, 30.3696) projected
  arc A7 (5.2891, 30.3696) -> (-39.7776, -7.802) centre (16.5131, -28.5713) ccw projected
  arc A8 (-44.4685, -11.0713) -> (-39.7776, -7.802) centre (-44.4685, -6.0713) ccw projected
  line L2 (-44.4685, -11.0713) -> (-68.4869, -11.0713) projected
  arc A9 (-68.4869, -11.0713) -> (-73.4869, -16.0713) centre (-68.4869, -16.0713) ccw projected
  line L3 (-73.4869, -16.0713) -> (-73.4869, -25.7717) projected
  ellipse E0 centre (-90.0533, -28.5713) end of major axis (-126.1955, -28.5713) minor radius 3.15 (-53.9112, -28.5713) -> (-73.4869, -25.7717) ccw projected
  line L4 (-53.9112, -28.5713) -> (-18.4869, -28.5713) projected
  arc A10 (-18.4869, -28.5713) -> (24.56, -62.6337) centre (16.5131, -28.5713) ccw projected
  line L5 (24.56, -62.6337) -> (11.2977, -85.6046) projected
  line L6 (11.2977, -85.6046) -> (-30.2715, -61.6046) projected
  arc A11 (-38.6208, -44.0713) -> (-30.2715, -61.6046) centre (16.5131, -28.5713) ccw projected
  line L7 (-38.6208, -44.0713) -> (-68.4869, -44.0713) projected
  line L8 (-68.4869, -44.0713) -> (-71.4869, -41.2625) projected
  line L9 (-71.4869, -41.2625) -> (-71.4869, -31.2739) projected
  ellipse E1 centre (-90.0533, -28.5713) end of major axis (-126.1955, -28.5713) minor radius 3.15 (-73.4869, -31.3709) -> (-71.4869, -31.2739) ccw projected
  line L10 (-73.4869, -31.3709) -> (-73.4869, -41.0713) projected
  arc A12 (-73.4869, -41.0713) -> (-68.4869, -46.0713) centre (-68.4869, -41.0713) ccw projected
  line L11 (-68.4869, -46.0713) -> (-44.4685, -46.0713) projected
  arc A13 (-39.7776, -49.3405) -> (-44.4685, -46.0713) centre (-44.4685, -51.0713) ccw projected
  arc A14 (-39.7776, -49.3405) -> (27.7371, 30.3696) centre (16.5131, -28.5713) ccw projected
  circle A15 centre (16.5131, -28.5713) radius 24
  arc A16 (45.5131, 21.6582) -> (27.7371, 28.3323) centre (16.5131, -28.5713) ccw projected
  line L12 (45.5131, 21.6582) -> (41.5131, 14.73) projected
  arc A17 (41.5131, 14.73) -> (-8.4869, 14.73) centre (16.5131, -28.5713) ccw projected
  line L13 (-8.4869, 14.73) -> (-12.4869, 21.6582) projected
  arc A18 (5.2891, 28.3323) -> (-12.4869, 21.6582) centre (16.5131, -28.5713) ccw projected
  point P0 (0, 0)
  dimension "d62" = 48
  constraints: 1 centre point, 1 coincident, 2 other
  measures "d62" diameter of A15
extrude "Extrusion16" cut sketch "Sketch16" against normal through all contours A15
body "Solid1"
